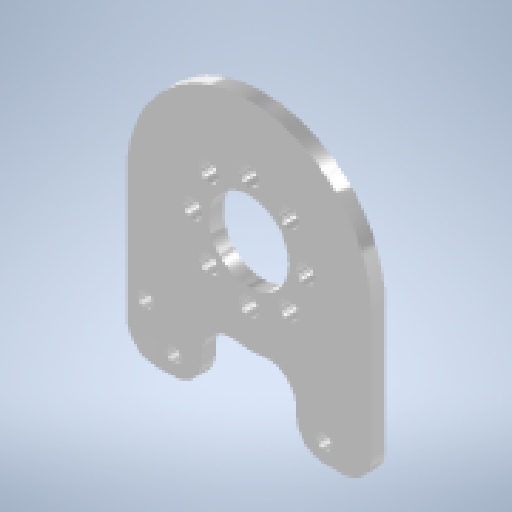
# Autodesk Inventor part: hipjoint_toleg_upper
Saved by Autodesk Inventor 2024.1 (Build 281209000, 209)
## iProperties
Created: 2024-02-12
Part Number: hipjoint_toleg_upper
Material: アルミニウム 6061
Document SubType Name: Modeling
Designer: hibik
Density: 2.7 g/cm^3
Appearance: アルミニウム - フラット
Author: hibik
Autodesk Inventor part; units mm, degrees
ref_plane "YZ Plane" through (0, 0, 0) normal (1, 0, 0) x (0, 1, 0)
ref_plane "XZ Plane" through (0, 0, 0) normal (0, 1, 0) x (-1, 0, 0)
ref_plane "XY Plane" through (0, 0, 0) normal (0, 0, 1) x (1, 0, 0)
sketch "スケッチ1" plane through (0, 0, 0) normal (0, 0, 1) x (1, 0, 0)
  line L0 (0, 16.5) -> (26, 16.5)
  line L1 (26, 16.5) -> (26, 0)
  line L2 (26, 0) -> (0, 0)
  line L3 (0, 0) -> (0, 16.5)
  circle A0 centre (13, 16.5) radius 13
  circle A1 centre (13, 16.5) radius 4.25
  circle A2 centre (13, 16.5) radius 6
  circle A3 centre (13, 22.5) radius 1
  circle A4 centre (8.7574, 20.7426) radius 1
  circle A5 centre (7, 16.5) radius 1
  circle A6 centre (8.7574, 12.2574) radius 1
  circle A7 centre (13, 10.5) radius 1
  circle A8 centre (17.2426, 12.2574) radius 1
  circle A9 centre (19, 16.5) radius 1
  circle A10 centre (17.2426, 20.7426) radius 1
  point P0 (0, 16.5)
  point P1 (26, 16.5)
  dimension "d3" = 12
  dimension "d0" = 16.5
  dimension "d1" = 26
  dimension "d2" = 8.5
  dimension "d4" = 2
  dimension "d7" = 360
  constraints: 10 centre point, 8 end point, 5 coincident, 2 midpoint, 2 parallel, 2 tangent, 2 vertical alignment, 1 horizontal, 1 perpendicular, 25 other
  measures "d0" distance of L2.end L0.start
  measures "d1" diameter of A0
  measures "d2" diameter of A1
  measures "d4" diameter of A3
extrude "押し出し1" add sketch "スケッチ1" along normal blind 1.5 contours A9 A2 A10 A3 A4 A5 L0 A0 | L0 A0 A5 A2 A6 A7 A8 A9 | A9 A2 A8 A7 A6 A5 L0 A1 | L0 A1 A5 A2 A4 A3 A10 A9 | L1 L2 L3 A0
sketch "スケッチ2" plane through (0, 0, 1.5) normal (0, 0, 1) x (1, 0, 0)
  circle A0 centre (2, 5.5906) radius 0.8 projected
  circle A1 centre (5, 2) radius 0.8 projected
  circle A2 centre (21, 2) radius 0.8 projected
  circle A3 centre (13, 16.5) radius 4.25 projected
  circle A4 centre (13, 16.5) radius 10
  line L0 (0, 0) -> (26, 0) projected
  line L1 (8, 7.8397) -> (8, 0)
  line L2 (18, 7.8397) -> (18, 0)
  point P0 (2, 0)
  point P1 (24, 0)
  dimension "d14" = 20
  dimension "d16" = 3
  dimension "d17" = 3
  constraints: 4 end point, 2 point on circle, 2 point on line, 1 centre point, 1 coincident, 1 perpendicular, 1 vertical
  measures "d14" diameter of A4
  measures "d16" distance from line of L1 A1.centre
  measures "d17" distance from line of A2.centre L2
extrude "押し出し2" cut sketch "スケッチ2" against normal through all contours A0 | A1 | A2 | A4 L2 L0 L1
fillet "フィレット2" radius 3 6 edges at (0, 0, 0.75) (8, 0, 0.75) (8, 7.8397, 0.75) (18, 7.8397, 0.75) (18, 0, 0.75) (26, 0, 0.75)
